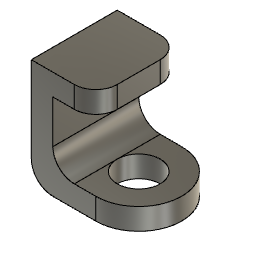
Exercise 3 (Autodesk Fusion 360 design; units mm, degrees)
Autodesk Fusion 360 part; units mm, degrees
sketch "Sketch1" plane through (0, 0, 0) normal (0, 1, 0) x (1, 0, 0)
  line L0 (0, -10) -> (0, -50.06)
  line L1 (0, -50.06) -> (30, -50.06)
  line L2 (30, -50.06) -> (30, -40.06)
  line L3 (30, -40.06) -> (10, -40.06)
  line L4 (10, 0) -> (50, 0)
  line L5 (50, 0) -> (50, -10)
  line L6 (50, -10) -> (20, -10)
  line L7 (10, -20) -> (10, -40.06)
  arc A0 (20, -10) -> (10, -20) centre (20, -20) ccw
  arc A1 (10, 0) -> (0, -10) centre (10, -10) ccw
  dimension "d1" = 50.06
  dimension "d2" = 30
  dimension "d3" = 10
  dimension "d4" = 20
  dimension "d6" = 50
  dimension "d7" = 10
  dimension "d8" = 10
  constraint vertical L0
  constraint perpendicular L0 L1
  constraint perpendicular L1 L2
  constraint perpendicular L2 L3
  constraint perpendicular L0 L4
  constraint perpendicular L4 L5
  constraint perpendicular L0 L6
  constraint perpendicular L3 L7
  constraint tangent L7 A0
  constraint tangent L6 A0
  constraint coincident origin L4
  constraint coincident origin L0
  constraint tangent L4 A1
  constraint tangent L0 A1
  measures "d1" distance of origin L0.end
  measures "d2" distance of L0.end L1.end
  measures "d3" distance of L1.end L2.end
  measures "d4" distance of L2.end L3.end
  measures "d6" distance of origin L4.end
  measures "d7" radius of A0
  measures "d8" radius of A1
extrude "Extrude1" add sketch "Sketch1" along normal blind 40
sketch "Sketch2" plane through (0, 0, 50.06) normal (0, 0, 1) x (-1, 0, 0)
  line L0 (0, 0) -> (-30, 0)
  line L1 (-30, 0) -> (-30, -40)
  line L2 (-30, -40) -> (0, -40)
  line L3 (0, -40) -> (0, 0)
  line L4 (0, -40) -> (-20, -40)
  line L5 (-30, -10) -> (-30, -30)
  line L6 (-20, 0) -> (0, 0)
  arc A0 (-30, -30) -> (-20, -40) centre (-20, -30) ccw
  arc A1 (-20, 0) -> (-30, -10) centre (-20, -10) ccw
  dimension "d11" = 10
  dimension "d12" = 10
  constraint coincident L2.end L3.start
  constraint coincident L0.start L3.end
  constraint tangent L4 A0
  constraint tangent L5 A0
  constraint tangent L5 A1
  constraint tangent L6 A1
  measures "d11" radius of A0
  measures "d12" radius of A1
extrude "Extrude2" cut sketch "Sketch2" against normal blind 10 contours L0 L1 A1 | L1 L2 A0
sketch "Sketch3" plane through (0, 0, 10) normal (0, 0, 1) x (-1, 0, 0)
  line L0 (-20, 0) -> (-50, 0)
  line L1 (-50, 0) -> (-50, -40)
  line L2 (-50, -40) -> (-20, -40)
  line L3 (-20, -40) -> (-20, 0)
  line L4 (-20, -40) -> (-30, -40)
  line L5 (-50, -20) -> (-50, -20)
  line L6 (-30, 0) -> (-20, 0)
  arc A0 (-50, -20) -> (-30, -40) centre (-30, -20) ccw
  arc A1 (-30, 0) -> (-50, -20) centre (-30, -20) ccw
  circle A2 centre (-30, -20) radius 10
  dimension "d15" = 20
  dimension "d16" = 20
  dimension "d17" = 20
  constraint coincident L2.end L3.start
  constraint coincident L0.start L3.end
  constraint tangent L4 A0
  constraint tangent L6 A1
  constraint concentric A1 A2
  measures "d15" radius of A0
  measures "d16" radius of A1
  measures "d17" diameter of A2
extrude "Extrude3" cut sketch "Sketch3" against normal blind 15 contours A2 | L0 L1 A1 | L1 L2 A0
